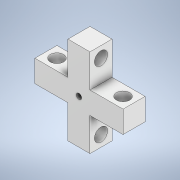
# Autodesk Inventor part: シリンダ先端パーツ
Saved by Autodesk Inventor 2021 (Build 250183000, 183)
## iProperties
Created: 2021-10-09
Part Number: シリンダ先端パーツ
Material: 一般
Document SubType Name: Modeling
Designer: ryusei
Density: 1 g/cm^3
Appearance: 滑らか - 白
Author: ryusei
Autodesk Inventor part; units mm, degrees
ref_plane "YZ Plane" through (0, 0, 0) normal (1, 0, 0) x (0, 1, 0)
ref_plane "XZ Plane" through (0, 0, 0) normal (0, 1, 0) x (-1, 0, 0)
ref_plane "XY Plane" through (0, 0, 0) normal (0, 0, 1) x (1, 0, 0)
sketch "スケッチ1" plane through (0, 0, 0) normal (0, 0, 1) x (1, 0, 0)
  line L0 (0, 0) -> (40, 0)
  line L1 (40, 0) -> (40, 40)
  line L2 (40, 40) -> (0, 40)
  line L3 (0, 40) -> (0, 0)
  dimension "d0" = 40
  dimension "d1" = 40
  constraints: 8 end point, 2 parallel, 1 horizontal, 1 perpendicular
  measures "d0" distance between parallel lines of L1 L3
  measures "d1" distance between parallel lines of L0 L2
extrude "押し出し1" add sketch "スケッチ1" along normal blind 10
sketch "スケッチ2" plane through (0, 0, 10) normal (0, 0, 1) x (1, 0, 0)
  line L0 (40, 40) -> (0, 40) projected
  line L1 (40, 40) -> (25, 40)
  line L2 (25, 40) -> (25, 25)
  line L3 (25, 25) -> (40, 25)
  line L4 (40, 25) -> (40, 40)
  point P0 (0, 0)
  point P1 (25, 40)
  dimension "d4" = 15
  dimension "d5" = 15
  constraints: 8 end point, 2 parallel, 1 horizontal, 1 perpendicular
  measures "d4" distance of L1.end L2.end
  measures "d5" distance of L2.end L3.end
extrude "押し出し2" cut sketch "スケッチ2" against normal blind 10
sketch "スケッチ3" plane through (0, 0, 10) normal (0, 0, 1) x (1, 0, 0)
  line L0 (0, 40) -> (15, 40)
  line L1 (15, 40) -> (15, 25)
  line L2 (15, 25) -> (0, 25)
  line L3 (0, 25) -> (0, 40)
  line L4 (0, 0) -> (40, 0) projected
  line L5 (0, 0) -> (15, 0)
  line L6 (15, 0) -> (15, 15)
  line L7 (15, 15) -> (0, 15)
  line L8 (0, 15) -> (0, 0)
  line L9 (40, 0) -> (25, 0)
  line L10 (25, 0) -> (25, 15)
  line L11 (25, 15) -> (40, 15)
  line L12 (40, 15) -> (40, 0)
  point P0 (25, 0)
  dimension "d8" = 15
  dimension "d9" = 15
  dimension "d10" = 15
  dimension "d11" = 15
  dimension "d12" = 15
  dimension "d13" = 15
  constraints: 24 end point, 6 parallel, 3 horizontal, 3 perpendicular
  measures "d8" distance of L1.end L2.end
  measures "d9" distance of L0.end L1.end
  measures "d10" distance of L6.end L7.end
  measures "d11" distance of L5.end L6.end
  measures "d12" distance of L9.end L10.end
  measures "d13" distance of L10.end L11.end
extrude "押し出し3" cut sketch "スケッチ3" against normal blind 10
sketch "スケッチ4" plane through (25, 25, 10) normal (1, 0, 0) x (0, 0, -1)
  line L0 (0, 15) -> (10, 15) projected
  line L1 (10, 15) -> (10, 0) projected
  line L2 (10, -10) -> (10, -25) projected
  line L3 (10, -25) -> (0, -25) projected
  point P0 (5, 10)
  point P1 (5, -20)
  dimension "d16" = 5
  dimension "d17" = 5
  dimension "d18" = 5
  dimension "d19" = 5
  measures "d16" distance from line of L0 point (5, 10)
  measures "d17" distance from line of L1 point (5, 10)
  measures "d18" distance from line of L2 point (5, -20)
  measures "d19" distance from line of L3 point (5, -20)
hole "穴1" at (25, 35, 5) at (25, 5, 5) direction (-1, 0, 0) diameter 6 end through all
sketch "スケッチ5" plane through (0, 25, 10) normal (0, 1, 0) x (1, 0, 0)
  line L0 (0, 10) -> (15, 10) projected
  line L1 (0, 0) -> (0, 10) projected
  line L2 (25, 10) -> (40, 10) projected
  line L3 (40, 10) -> (40, 0) projected
  point P0 (5, 5)
  point P1 (35, 5)
  dimension "d27" = 5
  dimension "d28" = 5
  dimension "d29" = 5
  dimension "d30" = 5
  measures "d27" distance from line of L0 point (5, 5)
  measures "d28" distance from line of L1 point (5, 5)
  measures "d29" distance from line of L2 point (35, 5)
  measures "d30" distance from line of L3 point (35, 5)
hole "穴2" at (5, 25, 5) at (35, 25, 5) direction (0, -1, 0) diameter 6 end through all
sketch "スケッチ6" plane through (0, 0, 10) normal (0, 0, 1) x (1, 0, 0)
  line L0 (40, 15) -> (40, 25) projected
  line L1 (25, 40) -> (15, 40) projected
  point P0 (0, 0)
  point P1 (20, 20)
  dimension "d38" = 20
  dimension "d39" = 20
  measures "d38" distance from line of L0 point (20, 20)
  measures "d39" distance from line of L1 point (20, 20)
hole "穴3" at (20, 20, 10) direction (0, 0, -1) diameter 2.459 end through all thread size "M3x0.5" class "6H" standard "ISO Metric profile"
